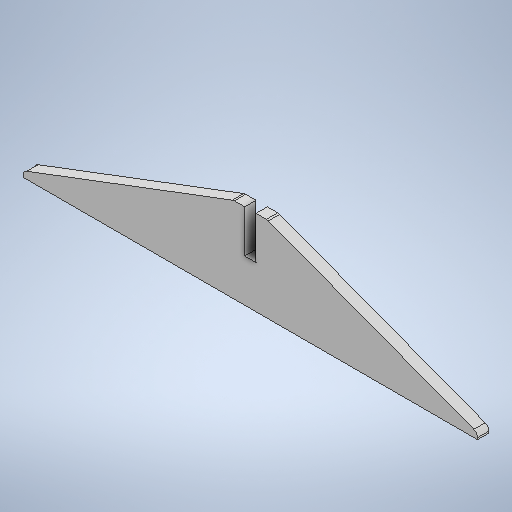
# Autodesk Inventor part: LegLessMaterial
Saved by Autodesk Inventor 2025.1 (Build 291241000, 241)
## iProperties
Created: 2025-03-30
Part Number: LegLessMaterial
Material: Všeobecné
Document SubType Name: Modeling
Designer: 42060
Density: 1 g/cm^3
Appearance: Výchozí
Author: 42060
Autodesk Inventor part; units mm, degrees
ref_plane "YZ Plane" through (0, 0, 0) normal (1, 0, 0) x (0, 1, 0)
ref_plane "XZ Plane" through (0, 0, 0) normal (0, 1, 0) x (-1, 0, 0)
ref_plane "XY Plane" through (0, 0, 0) normal (0, 0, 1) x (1, 0, 0)
sketch "Náčrt1" plane through (0, 0, 0) normal (0, 0, 1) x (1, 0, 0)
  line L0 (0, 15) -> (-2, 15)
  line L1 (-2, 15) -> (-2, 30)
  line L2 (-2, 30) -> (-5.6343, 30)
  line L3 (-6.3421, 29.8706) -> (-78.7078, 2.4889)
  line L4 (-80, 0.6184) -> (-80, 0)
  line L5 (-80, 0) -> (0, 0)
  arc A0 (-78.7078, 2.4889) -> (-80, 0.6184) centre (-78, 0.6184) ccw
  arc A1 (-5.6343, 30) -> (-6.3421, 29.8706) centre (-5.6343, 28) ccw
  line L6 (0, 15) -> (0, 0)
  line L7 (0, 15) -> (2, 15)
  line L8 (2, 15) -> (2, 30)
  line L9 (2, 30) -> (5.6343, 30)
  line L10 (6.3421, 29.8706) -> (78.7078, 2.4889)
  line L11 (80, 0.6184) -> (80, 0)
  line L12 (80, 0) -> (0, 0)
  arc A2 (80, 0.6184) -> (78.7078, 2.4889) centre (78, 0.6184) ccw
  arc A3 (6.3421, 29.8706) -> (5.6343, 30) centre (5.6343, 28) ccw
  point P0 (-6, 30)
  point P1 (-80, 2)
  point P2 (6, 30)
  point P3 (80, 2)
  dimension "d1" = 15
  dimension "d5" = 4
  dimension "d7" = 2
  dimension "d9" = 2
  dimension "d12" = 15
  dimension "d13" = 2
  dimension "d14" = 80
  constraints: 26 end point, 11 symmetric about line, 8 point on circle, 8 point on line, 4 centre point, 4 tangent, 2 perpendicular, 2 vertical, 1 equal radius, 1 horizontal, 1 parallel, 2 other
  measures "d1" distance between parallel lines of L5 L0
  measures "d5" distance of L1.end point (-6, 30)
  measures "d7" distance of point (-80, 2) L4.end
  measures "d9" radius of A0
  measures "d12" distance of L0.end L1.end
  measures "d13" distance of L0.start L0.end
  measures "d14" distance of L5.end L4.end
extrude "Vysunutí1" add sketch "Náčrt1" along normal mid plane 4
equation "\"d10\" = d4"
equation "\"d4\" = 4"
